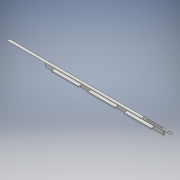
# Autodesk Inventor part: Roof Length Extension
Saved by Autodesk Inventor 2017 (Build 210142000, 142)
## iProperties
Created: 2018-03-29
Part Number: Roof Length Extension
Material: Generic
Document SubType Name: Modeling
Designer: Arjuna
Density: 1 g/cm^3
Appearance: Default
Author: Arjuna
## iProperties of the stored document Roof Length Extension_3DPrint.ipt
Created: 2018-03-30
Part Number: Roof Length Extension_3DPrint
Material: Generic
Document SubType Name: Modeling
Designer: Arjuna
Density: 1 g/cm^3
Appearance: Default
Author: Arjuna
Autodesk Inventor part; units mm, degrees
ref_plane "YZ Plane" through (0, 0, 0) normal (1, 0, 0) x (0, 1, 0)
ref_plane "XZ Plane" through (0, 0, 0) normal (0, 1, 0) x (-1, 0, 0)
sketch "Sketch2" plane through (0, 0, 0) normal (0, 0, 1) x (1, 0, 0)
  line L0 (-124.5, 2.5) -> (124.5, 2.5)
  line L1 (124.5, 2.5) -> (124.5, -2.5)
  line L2 (124.5, -2.5) -> (-124.5, -2.5)
  line L3 (-124.5, -2.5) -> (-124.5, 2.5)
  point P0 (0, 0)
  dimension "d1" = 249
  dimension "d2" = 5
  dimension "d3" = 2.5
  dimension "d4" = 124.5
  constraints: 8 end point, 2 parallel, 1 horizontal, 1 perpendicular
  measures "d1" distance of L1.end L2.end
  measures "d2" distance of L2.end L0.start
  measures "d3" vertical distance of point (0, 0) L0.start
  measures "d4" distance from line of point (0, 0) L3
sketch "Sketch3" plane through (0, 0, 0) normal (1, 0, 0) x (0, 1, 0)
  line L0 (0, 0) -> (-53.033, 53.033)
  line L1 (0, -0.5221) -> (1.6531, -0.5221)
  dimension "d5" = 75
  dimension "d6" = 45
  constraints: 4 end point, 1 horizontal
  measures "d5" distance of L0.start L0.end
  measures "d6" angle of L1 L0
sweep "Sweep1" add profiles "Sketch2" path "Sketch3" path curves L0
sketch "Sketch10" plane through (124.5, 2.5, 0) normal (0, 0, -1) x (-1, 0, 0)
  line L0 (249, 0) -> (0, 0) projected
  line L1 (0, 0) -> (0, -5) projected
  line L2 (0, -5) -> (249, -5) projected
  line L3 (249, -5) -> (249, 0) projected
  line L4 (15, 0) -> (234, 0)
  line L5 (234, 0) -> (234, -2)
  line L6 (234, -2) -> (15, -2)
  line L7 (15, -2) -> (15, 0)
  point P0 (124.5, -2.5)
  dimension "d76" = 2
  dimension "d77" = 219
  dimension "d78" = 109.5
  constraints: 8 end point, 2 parallel, 1 horizontal, 1 perpendicular, 1 point on line
  measures "d76" distance between parallel lines of L6 L0
  measures "d77" distance between parallel lines of L5 L7
  measures "d78" distance from line of point (124.5, -2.5) L7
extrude "Extrusion5" add sketch "Sketch10" along normal blind 10 contours L5 L6 L7 L0
sketch "Sketch11" plane through (-109.5, 0.5, 0) normal (0, -1, 0) x (1, 0, 0)
  line L0 (0, 0) -> (219, 0) projected
  line L1 (0, 0) -> (0, -10) projected
  line L2 (219, -10) -> (0, -10) projected
  line L3 (219, 0) -> (219, -10) projected
  line L4 (201.75, -6) -> (151.75, -6)
  line L5 (151.75, -6) -> (151.75, -4)
  line L6 (151.75, -4) -> (201.75, -4)
  line L7 (201.75, -4) -> (201.75, -6)
  line L8 (134.5, -6) -> (84.5, -6)
  line L9 (84.5, -6) -> (84.5, -4)
  line L10 (84.5, -4) -> (134.5, -4)
  line L11 (134.5, -4) -> (134.5, -6)
  line L12 (67.25, -6) -> (17.25, -6)
  line L13 (17.25, -6) -> (17.25, -4)
  line L14 (17.25, -4) -> (67.25, -4)
  line L15 (67.25, -4) -> (67.25, -6)
  point P0 (109.5, 0)
  dimension "d81" = 50
  dimension "d82" = 2
  dimension "d83" = 10
  dimension "d84" = 219
  dimension "d85" = 4
  dimension "d86" = 50
  dimension "d87" = 50
  dimension "d88" = 17.25
  dimension "d89" = 17.25
  dimension "d90" = 17.25
  dimension "d91" = 17.25
  constraints: 24 end point, 6 parallel, 4 point on line, 3 horizontal, 3 perpendicular
  measures "d81" distance of L4.start L4.end
  measures "d82" distance between parallel lines of L6 L4
  measures "d83" distance of L0.end L2.start
  measures "d84" distance of L2.start L1.end
  measures "d85" distance between parallel lines of L0 L6
  measures "d86" distance between parallel lines of L9 L11
  measures "d87" distance between parallel lines of L13 L15
  measures "d88" distance between parallel lines of L7 L3
  measures "d89" distance between parallel lines of L11 L5
  measures "d90" distance between parallel lines of L15 L9
  measures "d91" distance between parallel lines of L1 L13
extrude "Extrusion6" add sketch "Sketch11" along normal blind 6 contours L4 L5 L6 L7 | L8 L9 L10 L11 | L12 L13 L14 L15
sketch "Sketch13" plane through (124.5, -2.5, 0) normal (1, 0, 0) x (0, 0, -1)
  line L0 (0, 5) -> (0, 0) projected
  line L1 (0, 5) -> (-53.033, -48.033) projected
  line L2 (-53.033, -53.033) -> (-53.033, -48.033) projected
  line L3 (0, 0) -> (-53.033, -53.033) projected
  line L4 (-7.0711, -2.0711) -> (-7.0711, -4.5711)
  line L5 (-7.0711, -4.5711) -> (-45.9619, -43.4619)
  line L6 (-45.9619, -43.4619) -> (-45.9619, -40.9619)
  line L7 (-7.0711, -3.3211) -> (0, 3.75)
  line L8 (-45.9619, -42.2119) -> (-53.033, -49.283)
  point P0 (0, 2.5)
  dimension "d98" = 2.5
  dimension "d99" = 10
  dimension "d101" = 2.5
  dimension "d102" = 10
  dimension "d103" = 45
  constraints: 10 end point, 4 point on line, 3 parallel, 2 midpoint, 1 vertical
  measures "d98" distance of L4.start L4.end
  measures "d99" distance of L7.start L7.end
  measures "d101" distance of L5.end L6.end
  measures "d102" distance of L8.start L8.end
  measures "d103" angle of L6 L8
extrude "Extrusion7" cut sketch "Sketch13" against normal blind 10.5 contours L4 L5 L6 L1
ref_plane "Work Plane1" through (119.25, -2.5, 0) normal (1, 0, 0) x (0, 0, -1)
sketch "Sketch14" plane through (119.25, -2.5, 0) normal (1, 0, 0) x (0, 0, -1)
  line L0 (-7.0711, -2.0711) -> (-7.0711, -4.5711) projected
  line L1 (-7.0711, -4.5711) -> (-45.9619, -43.4619) projected
  line L2 (-45.9619, -43.4619) -> (-45.9619, -40.9619) projected
  line L3 (-45.9619, -40.9619) -> (-53.033, -48.033) projected
  line L4 (-53.033, -53.033) -> (-53.033, -48.033) projected
  line L5 (0, 0) -> (-53.033, -53.033) projected
  line L6 (0, 5) -> (0, 0) projected
  line L7 (0, 5) -> (-7.0711, -2.0711) projected
  line L8 (-45.9619, -40.9619) -> (-7.0711, -2.0711) projected
  line L9 (-45.9619, -43.4619) -> (-45.9619, -40.9619) projected
  line L10 (-7.0711, -4.5711) -> (-45.9619, -43.4619) projected
  line L11 (-7.0711, -2.0711) -> (-7.0711, -4.5711) projected
  line L12 (-13.0815, -10.5815) -> (-13.0815, -13.0815)
  line L13 (-23.6881, -21.1881) -> (-23.6881, -23.6881)
  line L14 (-29.3449, -26.8449) -> (-29.3449, -29.3449)
  line L15 (-39.9515, -37.4515) -> (-39.9515, -39.9515)
  line L16 (-23.6881, -21.1881) -> (-13.0815, -10.5815)
  line L17 (-13.0815, -13.0815) -> (-23.6881, -23.6881)
  line L18 (-29.3449, -26.8449) -> (-39.9515, -37.4515)
  line L19 (-29.3449, -29.3449) -> (-39.9515, -39.9515)
  line L20 (-39.9515, -39.9515) -> (-39.9515, -37.4515)
  line L21 (-39.9515, -37.4515) -> (-29.3449, -26.8449)
  line L22 (-29.3449, -26.8449) -> (-29.3449, -29.3449)
  line L23 (-29.3449, -29.3449) -> (-39.9515, -39.9515)
  line L24 (-23.6881, -21.1881) -> (-13.0815, -10.5815)
  line L25 (-13.0815, -10.5815) -> (-13.0815, -13.0815)
  line L26 (-13.0815, -13.0815) -> (-23.6881, -23.6881)
  line L27 (-23.6881, -23.6881) -> (-23.6881, -21.1881)
  point P0 (0, 2.5)
  dimension "d106" = 15
  dimension "d107" = 15
  dimension "d109" = 55
  dimension "d110" = 8.5
  dimension "d111" = 8.5
  dimension "d112" = 8
  constraints: 32 end point, 10 collinear, 8 point on line, 5 parallel, 1 vertical
  measures "d106" distance of L12.end L13.end
  measures "d107" distance of L14.end L15.end
  measures "d109" distance of L8.start L8.end
  measures "d110" distance of L0.end L12.start
  measures "d111" distance of L15.start L1.end
  measures "d112" distance of L13.end L14.end
extrude "Extrusion8" cut sketch "Sketch14" along normal mid plane 3 contours L12 L5 L13 L1 | L1 L14 L5 L15
mirror "Mirror2" about plane through (0, 0, 0) normal (1, 0, 0) of "Extrusion8", "Extrusion7"
ref_plane "Work Plane2" through (-119.25, -2.5, 0) normal (1, 0, 0) x (0, 0, -1)
equation "\"d3\" = 0.5 * d2"
equation "\"d4\" = 0.5 * d1"
equation "\"d78\" = 0.5 * d77"
equation "\"d85\" = -0.5 * d82 + 0.5 * d83"
equation "\"d86\" = d81"
equation "\"d87\" = d81"
equation "\"d88\" = -0.75 * d81 + 0.25 * d84"
equation "\"d89\" = d88"
equation "\"d90\" = d88"
equation "\"d111\" = d110"
body "Solid1"
